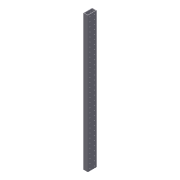
# Autodesk Inventor part: Conveyor_Frame_FrontTallRail_2x1
Saved by Autodesk Inventor 2012 (Build 160160000, 160)
## iProperties
Created: 2012-01-09
Part Number: Conveyor_Frame_FrontTallRail_2x1
Material: Aluminum-6061
Document SubType Name: Modeling
Designer: JesseK
Mass: 927.459 g
Surface Area: 2223.59 cm^2
Volume: 342.236 cm^3
Density: 2.71 g/cm^3
Author: JesseK
Autodesk Inventor part; units mm, degrees
ref_plane "YZ Plane" through (0, 0, 0) normal (1, 0, 0) x (0, 1, 0)
ref_plane "XZ Plane" through (0, 0, 0) normal (0, 1, 0) x (-1, 0, 0)
ref_plane "XY Plane" through (0, 0, 0) normal (0, 0, 1) x (1, 0, 0)
sketch "Sketch2" plane through (0, 0, 0) normal (0, 1, 0) x (-1, 0, 0)
  line L0 (0, 0) -> (25.4, 0)
  line L1 (25.4, 0) -> (25.4, 50.8)
  line L2 (25.4, 50.8) -> (0, 50.8)
  line L3 (0, 50.8) -> (0, 0)
  dimension "d0" = 25.4
  dimension "d1" = 50.8
  constraints: 8 end point, 2 parallel, 1 horizontal, 1 perpendicular
  measures "d0" distance of L1.end L2.end
  measures "d1" distance of L0.end L1.end
extrude "Extrusion1" add sketch "Sketch2" along normal blind 787.4
shell "Shell2" thickness 3.175 removed faces 2 at (-16.9333, 0, 16.9333) at (-16.9333, 787.4, 16.9333)
sketch "Sketch3" plane through (0, 0, 50.8) normal (1, 0, 0) x (0, 0, -1)
  line L0 (0, 0) -> (0, 787.4) projected
  line L1 (0, 0) -> (50.8, 0) projected
  circle A0 centre (12.7, 12.7) radius 2.3813
  dimension "d6" = 4.7625
  dimension "d7" = 12.7
  dimension "d8" = 12.7
  constraints: 1 centre point
  measures "d6" diameter of A0
  measures "d7" distance from line of L0 A0.centre
  measures "d8" distance from line of L1 A0.centre
extrude "Extrusion2" cut sketch "Sketch3" against normal through all
pattern_linear "Rectangular Pattern1" count 31 spacing 25.4 along (0, 1, 0) count 2 spacing 25.4 along (0, 0, -1) of "Extrusion2"
body "Solid1"
